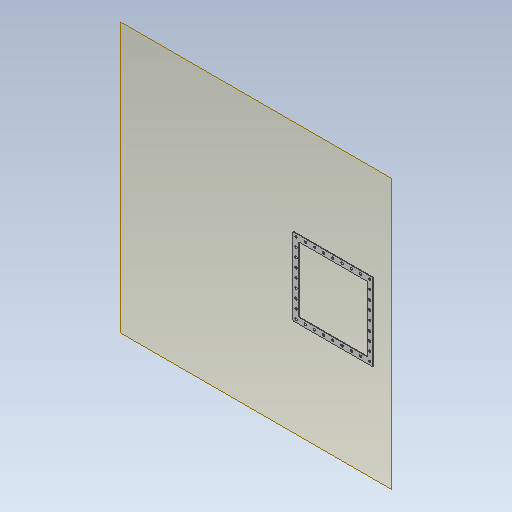
# Autodesk Inventor part: Прокладка рубашки охлаждения
Saved by Autodesk Inventor 2021 (Build 250183000, 183)
## iProperties
Created: 2020-11-15
Part Number: Прокладка рубашки охлаждения
Material: Типовые
Document SubType Name: Modeling
Designer: Тимоха
Density: 1 g/cm^3
Appearance: По умолчанию
Author: Тимоха
Autodesk Inventor part; units mm, degrees
ref_plane "YZ Plane" through (0, 0, 0) normal (1, 0, 0) x (0, 1, 0)
ref_plane "XZ Plane" through (0, 0, 0) normal (0, 1, 0) x (-1, 0, 0)
ref_plane "XY Plane" through (0, 0, 0) normal (0, 0, 1) x (1, 0, 0)
ref_plane "РабПлоскость1" through (-270.6167, -11.8042, 150.75) normal (0, 0, 1) x (1, 0, 0)
sketch "Эскиз1" plane through (-270.6167, -11.8042, 150.75) normal (0, 0, 1) x (1, 0, 0)
  circle A0 centre (393.9807, -108.1958) radius 4 projected
  circle A1 centre (393.9807, -78.1958) radius 4 projected
  circle A2 centre (393.9807, -48.1958) radius 4 projected
  circle A3 centre (393.9807, -18.1958) radius 4 projected
  circle A4 centre (393.9807, 11.8042) radius 4 projected
  circle A5 centre (393.9807, 41.8042) radius 4 projected
  circle A6 centre (393.9807, 71.8042) radius 4 projected
  circle A7 centre (393.9807, 101.8042) radius 4 projected
  circle A8 centre (393.9807, 131.8042) radius 4 projected
  circle A9 centre (362.9807, -108.1958) radius 4 projected
  circle A10 centre (362.9807, 131.8042) radius 4 projected
  circle A11 centre (331.9807, -108.1958) radius 4 projected
  circle A12 centre (331.9807, 131.8042) radius 4 projected
  circle A13 centre (300.9807, -108.1958) radius 4 projected
  circle A14 centre (300.9807, 131.8042) radius 4 projected
  circle A15 centre (269.9807, -108.1958) radius 4 projected
  circle A16 centre (269.9807, 131.8042) radius 4 projected
  circle A17 centre (238.9807, -108.1958) radius 4 projected
  circle A18 centre (238.9807, 131.8042) radius 4 projected
  circle A19 centre (207.9807, -108.1958) radius 4 projected
  circle A20 centre (207.9807, 131.8042) radius 4 projected
  circle A21 centre (176.9807, -108.1958) radius 4 projected
  circle A22 centre (176.9807, 131.8042) radius 4 projected
  circle A23 centre (145.9807, -108.1958) radius 4 projected
  circle A24 centre (145.9807, -78.1958) radius 4 projected
  circle A25 centre (145.9807, -48.1958) radius 4 projected
  circle A26 centre (145.9807, -18.1958) radius 4 projected
  circle A27 centre (145.9807, 11.8042) radius 4 projected
  circle A28 centre (145.9807, 41.8042) radius 4 projected
  circle A29 centre (145.9807, 71.8042) radius 4 projected
  circle A30 centre (145.9807, 101.8042) radius 4 projected
  circle A31 centre (145.9807, 131.8042) radius 4 projected
  line L0 (385.9807, 121.8042) -> (385.9807, -98.1958) projected
  line L1 (385.9807, -98.1958) -> (155.9807, -98.1958) projected
  line L2 (155.9807, -98.1958) -> (155.9807, 121.8042) projected
  line L3 (155.9807, 121.8042) -> (385.9807, 121.8042) projected
  arc A32 (137.9807, 141.8042) -> (135.9807, 139.8042) centre (137.9807, 139.8042) ccw projected
  line L4 (135.9807, 139.8042) -> (135.9807, -116.1958) projected
  arc A33 (135.9807, -116.1958) -> (137.9807, -118.1958) centre (137.9807, -116.1958) ccw projected
  line L5 (137.9807, -118.1958) -> (403.2527, -118.1958) projected
  arc A34 (403.2527, -118.1958) -> (405.2527, -116.1958) centre (403.2527, -116.1958) ccw projected
  line L6 (405.2527, -116.1958) -> (405.2527, 139.8042) projected
  arc A35 (405.2527, 139.8042) -> (403.2527, 141.8042) centre (403.2527, 139.8042) ccw projected
  line L7 (403.2527, 141.8042) -> (137.9807, 141.8042) projected
  point P0 (270.6167, 11.8042)
extrude "Выдавливание1" add sketch "Эскиз1" along normal blind 2
